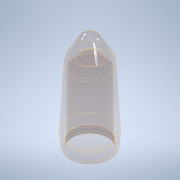
# Autodesk Inventor part: Upper
Saved by Autodesk Inventor 2021 (Build 250183000, 183)
## iProperties
Created: 2021-08-11
Part Number: Upper
Material: Polycarbonate, Smoke
Document SubType Name: Modeling
Designer: incep
Density: 1.2 g/cm^3
Appearance: Polycarbonate - Smoked
Author: incep
Autodesk Inventor part; units mm, degrees
ref_plane "YZ Plane" through (0, 0, 0) normal (1, 0, 0) x (0, 1, 0)
ref_plane "XZ Plane" through (0, 0, 0) normal (0, 1, 0) x (-1, 0, 0)
ref_plane "XY Plane" through (0, 0, 0) normal (0, 0, 1) x (1, 0, 0)
sketch "Bulb Copy" plane through (0, 0, 0) normal (0, 0, 1) x (1, 0, 0)
  line L0 (-16.5, 55) -> (16.5, 55) construction
  line L1 (16.5, 55) -> (16.5, 0)
  line L2 (16.5, 0) -> (-16.5, 0)
  line L3 (-16.5, 0) -> (-16.5, 55)
  line L4 (-10.5, 63) -> (10.5, 63)
  line L5 (10.5, 63) -> (10.5, 55) construction
  line L6 (10.5, 55) -> (-10.5, 55) construction
  line L7 (-10.5, 55) -> (-10.5, 63) construction
  line L8 (-16.5, 55) -> (-10.5, 63)
  line L9 (10.5, 63) -> (16.5, 55)
  line L10 (0, 63) -> (0, 0)
  point P0 (0, 55)
  dimension "d0" = 33
  dimension "d1" = 55
  dimension "d2" = 21
  dimension "d3" = 63
  constraints: 22 end point, 4 parallel, 2 horizontal, 2 midpoint, 2 perpendicular, 1 collinear, 1 vertical, 1 vertical alignment
  measures "d0" distance of L1.end L2.end
  measures "d1" distance of L0.end L1.end
  measures "d2" distance of L4.start L4.end
  measures "d3" distance from line of L10.end L4
sketch "Top Sketch" plane through (0, 0, 0) normal (0, 0, 1) x (1, 0, 0)
  line L0 (-17.5, 56) -> (17.5, 56) construction
  line L1 (17.5, 56) -> (17.5, -15) construction
  line L2 (17.5, -15) -> (-17.5, -15) construction
  line L3 (-17.5, -15) -> (-17.5, 56) construction
  line L4 (16.5, 55) -> (16.5, 0) projected
  line L5 (-16.5, 0) -> (-16.5, 55) projected
  line L6 (-19.5, 58) -> (19.5, 58) construction
  line L7 (19.5, 58) -> (19.5, -15) construction
  line L8 (19.5, -15) -> (-19.5, -15) construction
  line L9 (-19.5, -15) -> (-19.5, 58) construction
  line L10 (-22.5, 61) -> (22.5, 61) construction
  line L11 (22.5, 61) -> (22.5, -15) construction
  line L12 (22.5, -15) -> (-22.5, -15) construction
  line L13 (-22.5, -15) -> (-22.5, 61) construction
  line L14 (-10.5, 63) -> (10.5, 63) projected
  line L15 (-16.5, 55) -> (16.5, 55) construction
  line L16 (-22.5, 0) -> (-19.1379, 65) construction
  line L17 (22.5, 0) -> (19.1379, 65) construction
  line L18 (-19.1379, 65) -> (19.1379, 65) construction
  line L19 (-19.1379, 65) -> (0, 97.878) construction
  line L20 (0, 97.878) -> (19.1379, 65) construction
  line L21 (-16.5, 55) -> (-10.5, 63) projected
  line L22 (-22.4694, 0.5911) -> (-19.3883, 60.1601)
  line L23 (-16.6999, 69.1884) -> (-8.6425, 83.0307)
  line L24 (8.6425, 83.0307) -> (16.6999, 69.1884)
  line L25 (19.3883, 60.1601) -> (22.4694, 0.5911)
  arc A0 (-16.6999, 69.1884) -> (-19.3883, 60.1601) centre (0.585, 59.127) ccw
  arc A1 (19.3883, 60.1601) -> (16.6999, 69.1884) centre (-0.585, 59.127) ccw
  arc A2 (8.6425, 83.0307) -> (-8.6425, 83.0307) centre (0, 78) ccw
  line L26 (-22.4606, -0.5906) -> (-21.7499, -11.251)
  line L27 (22.4606, -0.5906) -> (21.5, -15)
  arc A3 (-22.4694, 0.5911) -> (-22.4606, -0.5906) centre (-12.4828, 0.0746) ccw
  arc A4 (22.4606, -0.5906) -> (22.4694, 0.5911) centre (12.4828, 0.0746) ccw
  line L28 (-17.5, 56) -> (-11.0463, 64.605)
  line L29 (-10.75, 65) -> (10.75, 65) construction
  line L30 (11.0463, 64.605) -> (17.5, 56)
  line L31 (10.5, 63) -> (16.5, 55) projected
  line L32 (0, -15) -> (0, 88) construction
  line L33 (17.5, -8) -> (-17.5, -8)
  line L34 (-17.5, 56) -> (-17.5, -8)
  line L35 (17.5, 56) -> (17.5, -8)
  line L36 (0, 88) -> (0, -15)
  line L37 (10.75, 65) -> (0, 76.7219) construction
  line L38 (0, 76.7219) -> (-10.75, 65) construction
  line L39 (10.4163, 65.3639) -> (7.37, 68.6856)
  line L40 (-7.37, 68.6856) -> (-10.4163, 65.3639)
  arc A5 (11.0463, 64.605) -> (10.4163, 65.3639) centre (3.0463, 58.605) ccw
  arc A6 (-10.4163, 65.3639) -> (-11.0463, 64.605) centre (-3.0463, 58.605) ccw
  arc A7 (7.37, 68.6856) -> (-7.37, 68.6856) centre (0, 61.9267) ccw
  line L41 (-17, 0) -> (-17, -31.7952) construction
  line L42 (-17, -31.7952) -> (17, -31.7952) construction
  line L43 (17, -31.7952) -> (17, 0) construction
  line L44 (14.5, 12.1752) -> (-14.5, 12.1752) construction
  line L45 (6.5, 0) -> (-6.5, 0) construction
  line L46 (-6.5, 0) -> (-6.5, -30) construction
  line L47 (-6.5, -30) -> (6.5, -30) construction
  line L48 (6.5, -30) -> (6.5, 0) construction
  line L49 (-6.5, -30) -> (-18.8432, -17.6568) construction
  arc A8 (-21.7499, -11.251) -> (-20.7451, -15) centre (-11.7721, -10.5858) ccw
  line L50 (0, -15) -> (-20.7451, -15)
  point P0 (0, 0)
  point P1 (-21.5, -15)
  point P2 (0, -8)
  point P3 (0, 65)
  point P4 (0, 71.9267)
  point P5 (0, 0)
  point P6 (0, -10)
  point P7 (0, 0)
  point P8 (0, 12.1752)
  dimension "d4" = 1
  dimension "d5" = 2
  dimension "d6" = 3
  dimension "d7" = 15
  dimension "d9" = 1
  dimension "d10" = 2
  dimension "d11" = 3
  dimension "d13" = 2
  dimension "d14" = 20
  dimension "d15" = 20
  dimension "d16" = 10
  dimension "d17" = 1
  dimension "d18" = 1
  dimension "d19" = 10
  dimension "d20" = 10
  dimension "d22" = 8
  dimension "d39" = 33
  dimension "d42" = 10
  dimension "d43" = 10
  dimension "d44" = 10
  dimension "d45" = 34
  dimension "d46" = 29
  dimension "d56" = 88
  dimension "d64" = 13
  dimension "d65" = 30
  dimension "d66" = 10
  constraints: 90 end point, 27 point on line, 19 point on circle, 18 tangent, 11 parallel, 9 centre point, 7 collinear, 7 vertical alignment, 6 horizontal, 5 midpoint, 4 coincident, 4 perpendicular, 2 horizontal alignment
  measures "d4" distance between parallel lines of L1 L4
  measures "d5" distance between parallel lines of L7 L1
  measures "d6" distance between parallel lines of L11 L7
  measures "d7" distance of point (0, -15) point (0, 0)
  measures "d9" distance between parallel lines of L15 L0
  measures "d10" distance between parallel lines of L0 L6
  measures "d11" distance between parallel lines of L6 L10
  measures "d13" distance between parallel lines of L14 L18
  measures "d14" radius of A0
  measures "d15" radius of A1
  measures "d16" radius of A2
  measures "d17" distance of point (-21.5, -15) L12.end
  measures "d18" distance of L11.end L27.end
  measures "d19" radius of A3
  measures "d20" radius of A4
  measures "d22" vertical distance of point (0, 0) L33.start
  measures "d39" distance between parallel lines of L5 L4
  measures "d42" radius of A5
  measures "d43" radius of A6
  measures "d44" radius of A7
  measures "d45" distance of L43.end L41.start
  measures "d46" distance of L44.start L44.end
  measures "d56" distance of L32.end point (0, 0)
  measures "d64" distance of L46.end L47.end
  measures "d65" distance of L45.end L46.end
  measures "d66" radius of A8
revolve "Top" add sketch "Top Sketch" angle 360 about axis through (0, 88, 0) along (0, -1, 0) contours L22 A0 L23 A2 L36 A7 L40 A6 L28 L34 L33 L50 A8 L26 A3
sketch "Sketch6" plane through (0, -15, 0) normal (0, -1, 0) x (1, 0, 0)
  circle A0 centre (0, 0) radius 3.2051 construction
  constraints: 1 centre point, 1 coincident
hole "Hole3" at (0, -15, 0) direction (0, 1, 0) diameter 36.3762 depth 8 tip angle 118 thread size "M38x1.5" class "6H" standard "ANSI Metric M Profile"
chamfer "Chamfer1" distance 0.5 angle 45 2 edges at (-12.3744, -6.5865, -12.3744) (12.3744, -6.5865, 12.3744)
body "Solid2"
